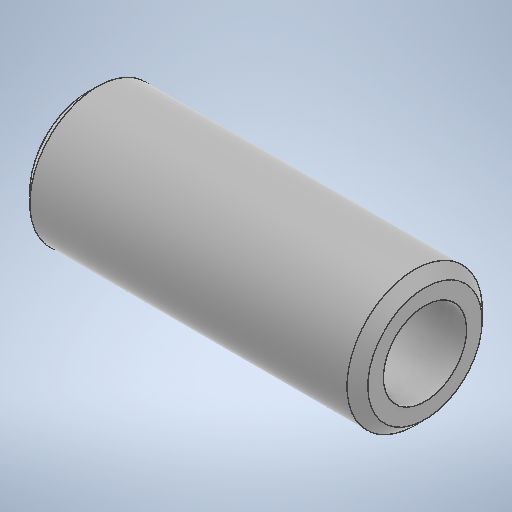
# Autodesk Inventor part: spacer_Φ3.2_1
Saved by Autodesk Inventor 2025 (Build 290162000, 162)
## iProperties
Created: 2025-09-16
Part Number: spacer_Φ3.2_1
Material: 一般
Document SubType Name: Modeling
Designer: sooo1
Density: 1 g/cm^3
Appearance: 滑らか - 標準の灰色
Author: sooo1
Autodesk Inventor part; units mm, degrees
ref_plane "YZ Plane" through (0, 0, 0) normal (1, 0, 0) x (0, 1, 0)
ref_plane "XZ Plane" through (0, 0, 0) normal (0, 1, 0) x (-1, 0, 0)
ref_plane "XY Plane" through (0, 0, 0) normal (0, 0, 1) x (1, 0, 0)
sketch "スケッチ1" plane through (0, 0, 0) normal (1, 0, 0) x (0, 1, 0)
  circle A0 centre (0, 0) radius 2.6
  circle A1 centre (0, 0) radius 1.6
  dimension "d0" = 3.2
  dimension "d1" = 1
  constraints: 2 centre point, 2 coincident
  measures "d0" diameter of A1
  measures "d1" radial gap between concentric circles of A1 A0
extrude "押し出し1" add sketch "スケッチ1" along normal mid plane 13
chamfer "面取り1" distance 0.4 angle 45 2 edges at (6.5, -2.6, 0) (-6.5, -2.6, 0)
